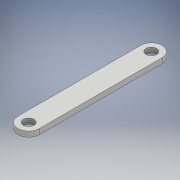
# Autodesk Inventor part: 連桿2
Saved by Autodesk Inventor 2017 (Build 210142000, 142)
## iProperties
Part Number: 連桿2
Material: 一般
Document SubType Name: Modeling
Designer: user
Density: 1 g/cm^3
Appearance: 預設
Author: user
Autodesk Inventor part; units mm, degrees
ref_plane "YZ Plane" through (0, 0, 0) normal (1, 0, 0) x (0, 1, 0)
ref_plane "XZ Plane" through (0, 0, 0) normal (0, 1, 0) x (-1, 0, 0)
ref_plane "XY Plane" through (0, 0, 0) normal (0, 0, 1) x (1, 0, 0)
sketch "草圖1" plane through (0, 0, 0) normal (0, 0, 1) x (1, 0, 0)
  line L0 (0, -11.505) -> (0, 11.505) construction
  line L1 (2, -11.505) -> (2, 11.505)
  line L2 (-2, 11.505) -> (-2, -11.505)
  arc A0 (-2, -11.505) -> (2, -11.505) centre (0, -11.505) ccw
  arc A1 (2, 11.505) -> (-2, 11.505) centre (0, 11.505) ccw
  point P0 (0, 0)
  dimension "d0" = 23.01
  dimension "d1" = 4
  constraints: 8 end point, 4 point on circle, 4 tangent, 2 centre point, 1 midpoint, 1 parallel, 1 vertical
  measures "d0" distance of L0.start L0.end
  measures "d1" distance between parallel lines of L2 L1
extrude "擠出1" add sketch "草圖1" along normal blind 1
sketch "草圖2" plane through (0, 0, 1) normal (0, 0, 1) x (1, 0, 0)
  arc A0 (2, 11.505) -> (-2, 11.505) centre (0, 11.505) ccw projected
  circle A1 centre (0, 11.505) radius 0.75
  arc A2 (-2, -11.505) -> (2, -11.505) centre (0, -11.505) ccw projected
  circle A3 centre (0, -11.505) radius 0.75
  point P0 (0, 0)
  dimension "d4" = 1.5
  dimension "d5" = 1.5
  constraints: 2 centre point, 2 coincident
  measures "d4" diameter of A1
  measures "d5" diameter of A3
extrude "擠出2" add sketch "草圖2" along normal blind 1
sketch "草圖3" plane through (0, 0, 1) normal (0, 0, 1) x (1, 0, 0)
  circle A0 centre (0, 11.505) radius 0.75 projected
  circle A1 centre (0, -11.505) radius 0.75 projected
  circle A2 centre (0, 11.505) radius 1
  circle A3 centre (0, -11.505) radius 1
  point P0 (0, 0)
  dimension "d8" = 2
  dimension "d9" = 2
  constraints: 2 centre point, 2 coincident
  measures "d8" diameter of A2
  measures "d9" diameter of A3
extrude "擠出3" cut sketch "草圖3" along normal mid plane 10 contours A0 | A1 | A2 | A3
